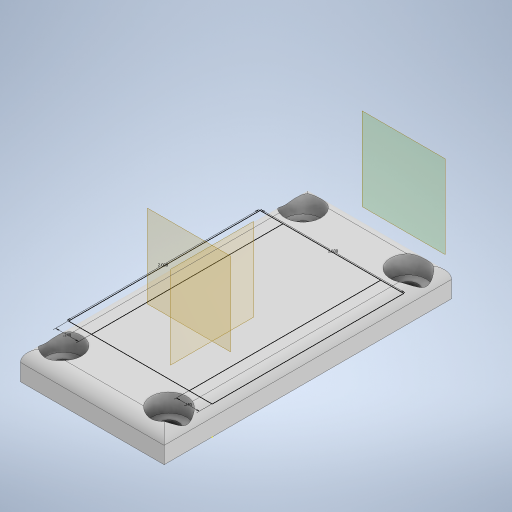
# Autodesk Inventor part: Sample Holder end for 8020-neutron-gen2
Saved by Autodesk Inventor 2024.1 (Build 281209000, 209)
## iProperties
Created: 2022-02-14
Part Number: Sample Holder end for 8020-neutron-gen2
Material: Generic
Document SubType Name: Modeling
Designer: Beaucage
Density: 1 g/cm^3
Appearance: Default
Author: Beaucage
Autodesk Inventor part; units mm, degrees
ref_plane "YZ Plane" through (0, 0, 0) normal (1, 0, 0) x (0, 1, 0)
ref_plane "XZ Plane" through (0, 0, 0) normal (0, 1, 0) x (-1, 0, 0)
ref_plane "XY Plane" through (0, 0, 0) normal (0, 0, 1) x (1, 0, 0)
sketch "Sketch1" plane through (0, 0, 0) normal (0, 1, 0) x (-1, 0, 0)
  line L0 (0, 0) -> (38.1, 0)
  line L1 (38.1, 0) -> (38.1, -50.8)
  line L2 (38.1, -50.8) -> (0, -50.8)
  line L3 (0, -50.8) -> (0, 0)
  line L4 (38.1, -50.8) -> (32.004, -50.8)
  line L5 (32.004, -50.8) -> (32.004, 0)
  line L6 (32.004, 0) -> (38.1, 0)
  line L7 (38.1, 0) -> (38.1, -50.8)
  line L8 (0, -50.8) -> (6.096, -50.8)
  line L9 (6.096, -50.8) -> (6.096, 0)
  line L10 (6.096, 0) -> (0, 0)
  line L11 (0, 0) -> (0, -50.8)
  dimension "d0" = 38.1
  dimension "d1" = 50.8
  dimension "d2" = 6.096
  dimension "d3" = 6.096
  constraints: 24 end point, 6 parallel, 3 horizontal, 3 perpendicular, 2 point on line
  measures "d0" distance of L1.end L2.end
  measures "d1" distance of L0.end L1.end
  measures "d2" distance of L5.end L6.end
  measures "d3" distance of L10.end L9.end
extrude "Extrusion2" add sketch "Sketch1" against normal blind 5.08
ref_plane "Work Plane1" through (0, 25.4, 0) normal (1, 0, 0) x (0, 0, -1)
ref_plane "Work Plane2" through (-6.096, 25.4, 0) normal (0, 0, 1) x (1, 0, 0)
ref_plane "Work Plane3" through (0, 25.4, -50.8) normal (0, 0, -1) x (-1, 0, 0)
sketch "Sketch3" plane through (-6.096, 25.4, 0) normal (0, 0, 1) x (1, 0, 0)
  line L0 (6.096, -30.48) -> (6.096, 0) projected
  line L1 (0, 0) -> (6.096, 0) projected
  line L2 (0, -25.4) -> (0, 0) projected
  line L3 (-25.908, -25.4) -> (0, -25.4) projected
  line L4 (-25.908, -25.4) -> (-25.908, 0) projected
  line L5 (-32.004, 0) -> (-25.908, 0) projected
  line L6 (-32.004, -30.48) -> (-32.004, 0) projected
  line L7 (6.096, -30.48) -> (-32.004, -30.48) projected
  line L8 (6.096, -25.4) -> (-32.004, -25.4) projected
  line L9 (6.096, -25.4) -> (-32.004, -25.4)
  constraints: 2 end point, 1 collinear
extrude "Extrusion3" add sketch "Sketch3" along normal blind 12.7 contours L7 L6 L8 L3 L0
sketch "Sketch4" plane through (0, 25.4, -50.8) normal (0, 0, -1) x (-1, 0, 0)
  line L0 (6.096, -25.4) -> (6.096, 0) projected
  line L1 (0, 0) -> (6.096, 0) projected
  line L2 (0, -30.48) -> (0, 0) projected
  line L3 (38.1, -30.48) -> (0, -30.48) projected
  line L4 (38.1, -30.48) -> (38.1, 0) projected
  line L5 (32.004, 0) -> (38.1, 0) projected
  line L6 (32.004, -25.4) -> (32.004, 0) projected
  line L7 (6.096, -25.4) -> (32.004, -25.4) projected
  line L8 (0, -25.4) -> (38.1, -25.4)
  constraints: 2 end point, 1 perpendicular, 1 point on line
extrude "Extrusion4" add sketch "Sketch4" along normal blind 12.7 contours L7 L8 L4 L3 L2
sketch "Sketch5" plane through (0, -5.08, 0) normal (0, -1, 0) x (1, 0, 0)
  line L0 (0, -63.5) -> (-38.1, -63.5) projected
  line L1 (-38.1, -63.5) -> (-38.1, 12.7) projected
  line L2 (0, 12.7) -> (0, -63.5) projected
  line L3 (-38.1, 12.7) -> (0, 12.7) projected
  line L4 (-26.924, -50.038) -> (-11.176, -50.038)
  line L5 (-11.176, -50.038) -> (-11.176, 1.27)
  line L6 (-11.176, 1.27) -> (-26.924, 1.27)
  line L7 (-26.924, 1.27) -> (-26.924, -50.038)
  line L8 (-26.924, -50.038) -> (-11.176, 1.27) construction
  line L9 (-11.176, -50.038) -> (-26.924, 1.27) construction
  line L10 (-19.05, 1.27) -> (-6.35, 1.27)
  line L11 (-6.35, 1.27) -> (-6.35, -43.18)
  line L12 (-6.35, -43.18) -> (-19.05, -43.18)
  line L13 (-19.05, -43.18) -> (-19.05, 1.27)
  line L14 (-19.05, 1.27) -> (-31.75, 1.27)
  line L15 (-31.75, 1.27) -> (-31.75, -43.18)
  line L16 (-31.75, -43.18) -> (-19.05, -43.18)
  line L17 (-19.05, -43.18) -> (-19.05, 1.27)
  point P0 (0, 0)
  point P1 (-19.05, -24.384)
  point P2 (-26.924, -43.18)
  point P3 (-11.176, -43.18)
  dimension "d20" = 15.748
  dimension "d21" = 51.308
  dimension "d22" = 12.7
  dimension "d23" = 44.45
  dimension "d24" = 12.7
  constraints: 28 end point, 6 parallel, 3 horizontal, 3 midpoint, 3 perpendicular
  measures "d20" distance of L6.end L5.end
  measures "d21" distance of L5.end L4.end
  measures "d22" distance of L11.end L12.end
  measures "d23" distance of L10.end L11.end
  measures "d24" distance of L16.end L15.end
extrude "Extrusion5" add sketch "Sketch5" along normal blind 2.54
sketch "Sketch6" plane through (0, -7.62, 0) normal (0, -1, 0) x (1, 0, 0)
  point P0 (0, 0)
sketch "Sketch7" plane through (0, -7.62, 0) normal (0, -1, 0) x (1, 0, 0)
  line L0 (0, -63.5) -> (0, 12.7) projected
  line L1 (0, -63.5) -> (-5.08, -63.5)
  line L2 (-5.08, -63.5) -> (-5.08, -57.15)
  line L3 (-5.08, -57.15) -> (0, -57.15)
  line L4 (0, -57.15) -> (0, -63.5)
  line L5 (-38.1, 12.7) -> (-38.1, -63.5) projected
  line L6 (-38.1, -63.5) -> (-33.02, -63.5)
  line L7 (-33.02, -63.5) -> (-33.02, -57.15)
  line L8 (-33.02, -57.15) -> (-38.1, -57.15)
  line L9 (-38.1, -57.15) -> (-38.1, -63.5)
  line L10 (-38.1, 12.7) -> (-33.02, 12.7)
  line L11 (-33.02, 12.7) -> (-33.02, 6.35)
  line L12 (-33.02, 6.35) -> (-38.1, 6.35)
  line L13 (-38.1, 6.35) -> (-38.1, 12.7)
  line L14 (0, 12.7) -> (-5.08, 12.7)
  line L15 (-5.08, 12.7) -> (-5.08, 6.35)
  line L16 (-5.08, 6.35) -> (0, 6.35)
  line L17 (0, 6.35) -> (0, 12.7)
  point P0 (0, 0)
  dimension "d27" = 5.08
  dimension "d28" = 6.35
  dimension "d29" = 5.08
  dimension "d30" = 6.35
  dimension "d31" = 5.08
  dimension "d32" = 6.35
  dimension "d33" = 5.08
  constraints: 32 end point, 8 parallel, 4 horizontal, 4 perpendicular, 3 point on line
  measures "d27" distance of L2.end L3.end
  measures "d28" distance of L1.end L2.end
  measures "d29" distance of L8.end L7.end
  measures "d30" distance of L7.end L6.end
  measures "d31" distance of L11.end L12.end
  measures "d32" distance of L10.end L11.end
  measures "d33" distance of L16.end L15.end
hole "Hole2" at (-5.08, -7.62, -57.15) at (-33.02, -7.62, -57.15) at (-5.08, -7.62, 6.35) at (-33.02, -7.62, 6.35) direction (0, 1, 0) diameter 3.7973 end through all
sketch "Sketch8" plane through (0, 0, 0) normal (0, 1, 0) x (1, 0, 0)
  circle A0 centre (-33.02, -6.35) radius 1.8986 projected
  circle A1 centre (-5.08, -6.35) radius 1.8986 projected
  circle A2 centre (-5.08, 57.15) radius 1.8986 projected
  point P0 (0, 0)
  point P1 (-33.02, 57.15)
  constraints: 3 coincident
hole "Hole3" at (-33.02, 0, 6.35) at (-5.08, 0, 6.35) at (-33.02, 0, -57.15) at (-5.08, 0, -57.15) direction (0, -1, 0) diameter 5.1054 end through all counterbore diameter 9.525 counterbore depth 4.826 clearance for "Socket Head Cap Screw" size "#10" standard "Ansi Unified Screw Threads"
fillet "Fillet1" radius 3.175 4 edges at (0, 0, -25.4) (-19.05, 0, 12.7) (-38.1, 0, -25.4) (-19.05, 0, -63.5)
sketch "Sketch9" plane through (0, -7.62, 0) normal (0, -1, 0) x (1, 0, 0)
  line L0 (-6.35, 1.27) -> (-6.35, -43.18) projected
  line L1 (-6.35, 1.27) -> (-6.35, -3.048)
  line L2 (-31.75, 1.27) -> (-31.75, -43.18) projected
  line L3 (-31.75, 1.27) -> (-31.75, -3.048)
  line L4 (-6.35, -43.18) -> (-6.35, -38.862)
  line L5 (-6.35, -38.862) -> (-31.75, -38.862)
  line L6 (-8.89, 0.762) -> (-3.81, 0.762)
  line L7 (-3.81, 0.762) -> (-3.81, -6.858)
  line L8 (-3.81, -6.858) -> (-8.89, -6.858)
  line L9 (-8.89, -6.858) -> (-8.89, 0.762)
  line L10 (-8.89, 0.762) -> (-3.81, -6.858) construction
  line L11 (-3.81, 0.762) -> (-8.89, -6.858) construction
  line L12 (-8.89, -35.052) -> (-3.81, -35.052)
  line L13 (-3.81, -35.052) -> (-3.81, -42.672)
  line L14 (-3.81, -42.672) -> (-8.89, -42.672)
  line L15 (-8.89, -42.672) -> (-8.89, -35.052)
  line L16 (-8.89, -35.052) -> (-3.81, -42.672) construction
  line L17 (-3.81, -35.052) -> (-8.89, -42.672) construction
  line L18 (-34.29, -35.052) -> (-29.21, -35.052)
  line L19 (-29.21, -35.052) -> (-29.21, -42.672)
  line L20 (-29.21, -42.672) -> (-34.29, -42.672)
  line L21 (-34.29, -42.672) -> (-34.29, -35.052)
  line L22 (-34.29, -35.052) -> (-29.21, -42.672) construction
  line L23 (-29.21, -35.052) -> (-34.29, -42.672) construction
  line L24 (-34.29, 0.762) -> (-29.21, 0.762)
  line L25 (-29.21, 0.762) -> (-29.21, -6.858)
  line L26 (-29.21, -6.858) -> (-34.29, -6.858)
  line L27 (-34.29, -6.858) -> (-34.29, 0.762)
  line L28 (-34.29, 0.762) -> (-29.21, -6.858) construction
  line L29 (-29.21, 0.762) -> (-34.29, -6.858) construction
  point P0 (0, 0)
  dimension "d49" = 4.318
  dimension "d50" = 4.318
  dimension "d51" = 4.318
  dimension "d52" = 5.08
  dimension "d53" = 7.62
  dimension "d54" = 5.08
  dimension "d55" = 7.62
  dimension "d56" = 5.08
  dimension "d57" = 7.62
  constraints: 56 end point, 8 midpoint, 8 parallel, 6 point on line, 5 perpendicular, 4 horizontal
  measures "d49" distance of L0.start L1.end
  measures "d50" distance of L2.start L3.end
  measures "d51" distance of L0.end L4.end
  measures "d52" distance of L7.end L8.end
  measures "d53" distance of L6.end L7.end
  measures "d54" distance of L13.end L14.end
  measures "d55" distance of L12.end L13.end
  measures "d56" distance of L19.end L20.end
  measures "d57" distance of L18.end L19.end
extrude "Extrusion6" cut sketch "Sketch9" against normal up to surface (2.54 mm away)
body "Solid1"
